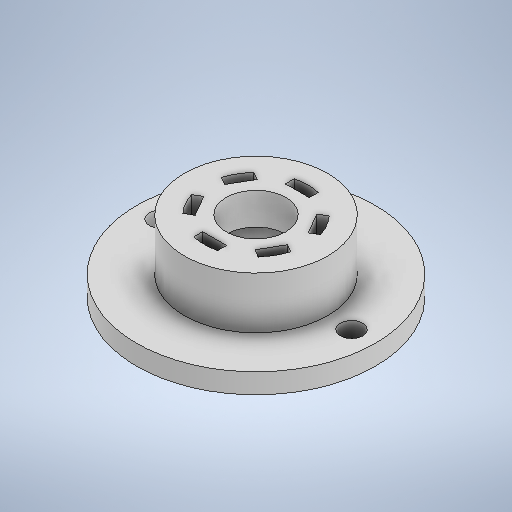
# Autodesk Inventor part: Potentiometer_Holder_Main
Saved by Autodesk Inventor 2025 (Build 290162000, 162)
## iProperties
Created: 2024-11-19
Part Number: Potentiometer_Holder_Main
Material: Generic
Document SubType Name: Modeling
Designer: phil
Density: 1 g/cm^3
Appearance: Default
Author: phil
Autodesk Inventor part; units mm, degrees
ref_plane "YZ Plane" through (0, 0, 0) normal (1, 0, 0) x (0, 1, 0)
ref_plane "XZ Plane" through (0, 0, 0) normal (0, 1, 0) x (-1, 0, 0)
ref_plane "XY Plane" through (0, 0, 0) normal (0, 0, 1) x (1, 0, 0)
sketch "Sketch1" plane through (0, 0, 0) normal (0, 1, 0) x (-1, 0, 0)
  circle A0 centre (0, 0) radius 3.75
  circle A1 centre (0, 0) radius 6.5
  circle A2 centre (0, 0) radius 9
  dimension "d0" = 7.5
  dimension "d1" = 13
  dimension "d2" = 2.5
  constraints: 3 centre point, 2 coincident
  measures "d0" diameter of A0
  measures "d1" diameter of A1
  measures "d2" radial gap between concentric circles of A1 A2
extrude "Extrusion1" add sketch "Sketch1" along normal blind 4 contours A1 | A2
extrude "Extrusion2" add sketch "Sketch1" against normal blind 5 contours A2
sketch "Sketch2" plane through (0, 0, 0) normal (0, -1, 0) x (1, 0, 0)
  circle A0 centre (0, 0) radius 6.5 projected
  circle A1 centre (0, 0) radius 3.75 projected
  circle A2 centre (0, 0) radius 9 projected
  circle A3 centre (0, 0) radius 6.5 projected
  line L0 (0, 6.5) -> (-1.5, 6.5)
  line L1 (-1.5, 6.5) -> (-1.5, 5.2)
  line L2 (-1.5, 5.2) -> (0, 5.2)
  line L3 (0, 5.2) -> (0, 6.5)
  line L4 (0, 6.5) -> (1.5, 6.5)
  line L5 (1.5, 6.5) -> (1.5, 5.2)
  line L6 (1.5, 5.2) -> (0, 5.2)
  arc A4 (1.5, 6.3246) -> (-1.5, 6.3246) centre (0, 0) ccw
  line L7 (-6.3792, 1.951) -> (-5.2533, 1.301)
  line L8 (-5.2533, 1.301) -> (-4.5033, 2.6)
  line L9 (-3.7533, 3.899) -> (-4.5033, 2.6)
  line L10 (-4.8792, 4.549) -> (-3.7533, 3.899)
  arc A5 (-4.7272, 4.4613) -> (-6.2272, 1.8632) centre (0, 0) ccw
  line L11 (-4.8792, -4.549) -> (-3.7533, -3.899)
  line L12 (-3.7533, -3.899) -> (-4.5033, -2.6)
  line L13 (-5.2533, -1.301) -> (-4.5033, -2.6)
  line L14 (-6.3792, -1.951) -> (-5.2533, -1.301)
  arc A6 (-6.2272, -1.8632) -> (-4.7272, -4.4613) centre (0, 0) ccw
  line L15 (1.5, -6.5) -> (1.5, -5.2)
  line L16 (1.5, -5.2) -> (0, -5.2)
  line L17 (-1.5, -5.2) -> (0, -5.2)
  line L18 (-1.5, -6.5) -> (-1.5, -5.2)
  arc A7 (-1.5, -6.3246) -> (1.5, -6.3246) centre (0, 0) ccw
  line L19 (6.3792, -1.951) -> (5.2533, -1.301)
  line L20 (5.2533, -1.301) -> (4.5033, -2.6)
  line L21 (3.7533, -3.899) -> (4.5033, -2.6)
  line L22 (4.8792, -4.549) -> (3.7533, -3.899)
  arc A8 (4.7272, -4.4613) -> (6.2272, -1.8632) centre (0, 0) ccw
  line L23 (4.8792, 4.549) -> (3.7533, 3.899)
  line L24 (3.7533, 3.899) -> (4.5033, 2.6)
  line L25 (5.2533, 1.301) -> (4.5033, 2.6)
  line L26 (6.3792, 1.951) -> (5.2533, 1.301)
  arc A9 (6.2272, 1.8632) -> (4.7272, 4.4613) centre (0, 0) ccw
  point P0 (-5.6292, 3.25)
  point P1 (-5.6292, -3.25)
  point P2 (0, -6.5)
  point P3 (5.6292, -3.25)
  point P4 (5.6292, 3.25)
  point P5 (-1.5, -6.3246)
  point P6 (1.5, -6.3246)
  point P7 (4.7272, -4.4613)
  point P8 (6.2272, -1.8632)
  point P9 (6.2272, 1.8632)
  point P10 (1.5, 6.3246)
  point P11 (-1.5, 6.3246)
  point P12 (-4.7272, 4.4613)
  point P13 (-6.2272, 1.8632)
  point P14 (-6.2272, -1.8632)
  dimension "d7" = 1.5
  dimension "d8" = 1.3
  dimension "d9" = 5.2
  dimension "d12" = 360
  constraints: 54 end point, 21 point on circle, 12 point on line, 6 centre point, 2 parallel, 2 symmetric about line, 1 horizontal, 1 perpendicular, 85 other
  measures "d7" distance of L2.end L1.end
  measures "d8" distance of L1.end L0.end
  measures "d9" distance of point (0, 0) L2.end
extrude "Extrusion3" cut sketch "Sketch2" against normal blind 4 contours L26 L25 L24 L23 A0 | A0 L22 L21 L20 L19 | L5 L6 L3 A0 | A0 L18 L17 L16 L15 | L3 L2 L1 A0 | A0 L14 L13 L12 L11 | L10 L9 L8 L7 A0
sketch "Sketch3" plane through (0, -5, 0) normal (0, -1, 0) x (1, 0, 0)
  circle A0 centre (0, 0) radius 15
  circle A1 centre (0, 0) radius 9 projected
  circle A2 centre (0, 0) radius 6.5 projected
  circle A3 centre (12, 0) radius 1.4
  circle A4 centre (-12, 0) radius 1.4
  dimension "d16" = 30
  dimension "d19" = 2.8
  dimension "d20" = 12
  dimension "d23" = 360
  constraints: 3 centre point, 3 coincident, 5 other
  measures "d16" diameter of A0
  measures "d19" diameter of A3
  measures "d20" distance of A0.centre A3.centre
extrude "Extrusion4" add sketch "Sketch3" against normal blind 2.5 contours A0
body "Solid1"
